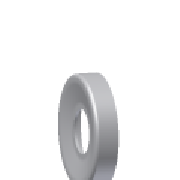
# Autodesk Inventor part: BrakeDrum
Saved by Autodesk Inventor 2016 (Build 200138000, 138)
## iProperties
Shininess: 86.0
Length Units: 11272
Angle Units: 11279
Time Units: 11290
Mass Units: 11286
Length Display Precision: 3
Angle Display Precision: 2
Compacted: True
Created: 2001-05-25
Part Number: BrakeDrum
Document SubType Name: Modeling
Designer: Administrator
Material: Generic
Density: 1 g/cm^3
Appearance: Chrome - Polished
Density: 0.0
Volumn: 0.0
Area: 0.0
PropertySet Name: Model Information
Control State: 0
Master: False
Checked Out: False
Author: Administrator
Autodesk Inventor part; units mm, degrees
ref_plane "YZ Plane" through (0, 0, 0) normal (1, 0, 0) x (0, 1, 0)
ref_plane "XZ Plane" through (0, 0, 0) normal (0, 1, 0) x (-1, 0, 0)
ref_plane "XY Plane" through (0, 0, 0) normal (0, 0, 1) x (1, 0, 0)
sketch "Sketch1" plane through (0, 0, 0) normal (0, 0, 1) x (1, 0, 0)
  line L0 (0, -8.1326) -> (0, 105.7239) projected
  line L1 (-30.6691, 0) -> (36.0366, 0) projected
  line L2 (0, 31.75) -> (0, 36.8263)
  arc A0 (0, 36.8263) -> (-0.8357, 43.3529) centre (-25.9044, 36.8263) ccw
  line L3 (-0.8357, 43.3529) -> (-6.8264, 66.3636)
  arc A1 (-7.531, 71.8662) -> (-6.8264, 66.3636) centre (14.3094, 71.8662) ccw
  line L4 (-7.531, 71.8662) -> (-7.531, 74.5808)
  arc A2 (-6.007, 76.1048) -> (-7.531, 74.5808) centre (-6.007, 74.5808) ccw
  line L5 (-6.007, 76.1048) -> (21.7425, 76.1048)
  line L6 (21.7425, 80.1688) -> (-6.007, 80.1688)
  arc A3 (-6.007, 80.1688) -> (-11.595, 74.5808) centre (-6.007, 74.5808) ccw
  line L7 (-11.595, 74.5808) -> (-11.595, 71.8662)
  arc A4 (-11.595, 71.8662) -> (-10.7593, 65.3396) centre (14.3094, 71.8662) ccw
  line L8 (-10.7593, 65.3396) -> (-4.7686, 42.329)
  arc A5 (-4.064, 36.8263) -> (-4.7686, 42.329) centre (-25.9044, 36.8263) ccw
  line L9 (-4.064, 36.8263) -> (-4.064, 31.75)
  line L10 (-4.064, 31.75) -> (0, 31.75)
  line L11 (21.7425, 80.1688) -> (21.7425, 76.1048)
  point P0 (0, 0)
  dimension "d0" = 33.3375
  dimension "d1" = 4.064
  dimension "d2" = 1.524
  dimension "d3" = 63.5
  dimension "d4" = 160.3375
  constraints: 20 end point, 12 point on circle, 12 tangent, 6 centre point, 3 perpendicular, 2 point on line, 1 equal radius, 1 parallel, 6 other
  measures "d0" distance from line of L6.start L7
  measures "d1" distance of L6.start L5.end
  measures "d2" radius of A2
  measures "d3" diameter of L10 L1
  measures "d4" diameter of L6 L1
revolve "Revolution1" add sketch "Sketch1" angle 360 about axis through (-10, 0, 0) along (1, 0, 0) contours L10 L9 A5 L8 A4 L7 A3 L6 L0 L5 A2 L4 A1 L3 A0 | L0 L6 L11 L5
body "Solid1"
